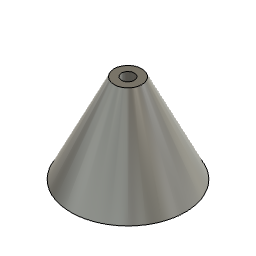
Piece_Conique v0 (Autodesk Fusion 360 design; units mm, degrees)
Autodesk Fusion 360 part; units mm, degrees
sketch "Esquisse1" plane through (0, 0, 0) normal (0, 1, 0) x (1, 0, 0)
  circle A0 centre (0, 0) radius 45
  dimension "d1" = 90
  constraint coincident A0.centre origin
  measures "d1" diameter of A0
sketch "Esquisse2" plane through (0, 0, 0) normal (0, 1, 0) x (1, 0, 0)
  circle A0 centre (0, 0) radius 43
  dimension "d2" = 86
  constraint coincident A0.centre origin
  measures "d2" diameter of A0
sketch "Esquisse3" plane through (0, 0, 0) normal (0, 1, 0) x (1, 0, 0)
  circle A0 centre (0, 0) radius 35.5
  dimension "d3" = 71
  constraint coincident A0.centre origin
  measures "d3" diameter of A0
extrude "Extrusion1" add sketch "Esquisse1" along normal blind 70 draft -26
sketch "Esquisse4" plane through (0, 70, 0) normal (0, 1, 0) x (-1, 0, 0)
  circle A0 centre (0, 0) radius 10.8587
  circle A1 centre (0, 0) radius 5
  dimension "d6" = 10
  constraint coincident A0.centre A1.centre
  measures "d6" diameter of A1
extrude "Extrusion2" cut sketch "Esquisse2" along normal blind 5 draft -26
extrude "Extrusion3" cut sketch "Esquisse4" against normal blind 15 contours A1
extrude "Extrusion4" cut sketch "Esquisse3" along normal blind 70 draft -26
sketch "Esquisse5" plane through (0, 0, 0) normal (0, 0, 1) x (1, 0, 0)
